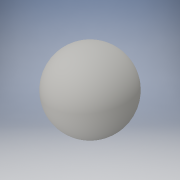
# Autodesk Inventor part: Basketball
Saved by Autodesk Inventor 2016 (Build 200138000, 138)
## iProperties
Created: 2015-09-29
Part Number: Basketball
Material: Generic
Document SubType Name: Modeling
Designer: Mack
Density: 1 g/cm^3
Appearance: Default
Author: Mack
Autodesk Inventor part; units mm, degrees
ref_plane "YZ Plane" through (0, 0, 0) normal (1, 0, 0) x (0, 1, 0)
ref_plane "XZ Plane" through (0, 0, 0) normal (0, 1, 0) x (-1, 0, 0)
ref_plane "XY Plane" through (0, 0, 0) normal (0, 0, 1) x (1, 0, 0)
sketch "Sketch1" plane through (0, 0, 0) normal (0, 0, 1) x (1, 0, 0)
  arc A0 (0, -141.4887) -> (0, 141.4887) centre (0, 0) ccw
  line L0 (0, 141.4887) -> (0, -141.4887)
  dimension "d0" = 282.9775
  dimension "d1" = 141.4887
  constraints: 2 end point, 2 point on circle, 1 centre point, 1 coincident, 1 vertical
  measures "d0" diameter of A0
  measures "d1" distance edge to line of A0 L0
revolve "Revolution1" add sketch "Sketch1" angle 360 about axis through (0, 141.4887, 0) along (0, -1, 0)
equation "\"d1\" = 0.5 * d0"
body "Solid1"
